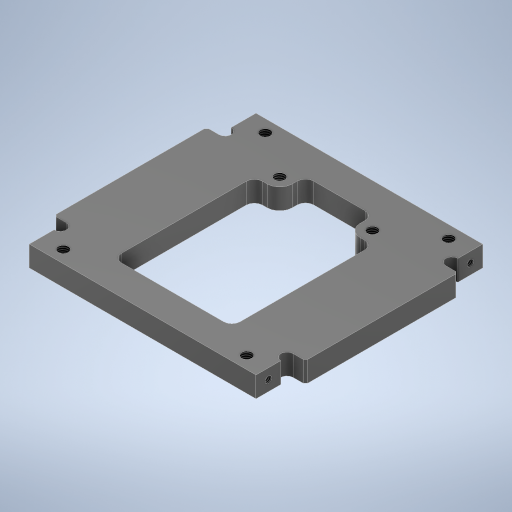
# Autodesk Inventor part: HeadUpperFrame
Saved by Autodesk Inventor 2024.2 (Build 282272000, 272)
## iProperties
Created: 2024-06-11
Part Number: HeadUpperFrame
Material: Acetal Resin, Black
Document SubType Name: Modeling
Designer: Masato Kubotera
Density: 1.425 g/cm^3
Appearance: Smooth - Black
Author: Masato Kubotera
Autodesk Inventor part; units mm, degrees
ref_plane "YZ Plane" through (0, 0, 0) normal (1, 0, 0) x (0, 1, 0)
ref_plane "XZ Plane" through (0, 0, 0) normal (0, 1, 0) x (-1, 0, 0)
ref_plane "XY Plane" through (0, 0, 0) normal (0, 0, 1) x (1, 0, 0)
sketch "Sketch1" plane through (0, 0, 0) normal (0, 0, 1) x (1, 0, 0)
  line L0 (-27.5, -27.5) -> (27.5, -27.5)
  line L1 (27.5, -27.5) -> (27.5, 27.5)
  line L2 (27.5, 27.5) -> (-27.5, 27.5)
  line L3 (-27.5, 27.5) -> (-27.5, -27.5)
  line L4 (-27.5, -27.5) -> (27.5, 27.5) construction
  line L5 (27.5, -27.5) -> (-27.5, 27.5) construction
  line L6 (-20, 14.15) -> (20, 14.15) construction
  line L7 (20, 14.15) -> (20, -14.15) construction
  line L8 (20, -14.15) -> (-20, -14.15) construction
  line L9 (-20, -14.15) -> (-20, 14.15) construction
  line L10 (-20, 14.15) -> (20, -14.15) construction
  line L11 (20, 14.15) -> (-20, -14.15) construction
  line L12 (0, -27.5) -> (0, 27.5) construction
  line L13 (-27.5, 0) -> (27.5, 0)
  line L14 (17, 11.25) -> (-17, 11.25) construction
  line L15 (-17, 11.25) -> (-17, -11.25) construction
  line L16 (-17, -11.25) -> (17, -11.25) construction
  line L17 (17, -11.25) -> (17, 11.25) construction
  line L18 (17, 11.25) -> (-17, -11.25) construction
  line L19 (-17, 11.25) -> (17, -11.25) construction
  line L20 (20.25, -12.4) -> (20.25, 12.4)
  line L21 (-18.5, -27.5) -> (-18.5, -30.5)
  line L22 (-18.5, -30.5) -> (18.5, -30.5)
  line L23 (18.5, -30.5) -> (18.5, -27.5)
  arc A0 (-18.5, -27.5) -> (-21.5, -27.5) centre (-20, -27.5) ccw
  line L24 (-24.5, -27.5) -> (-24.5, -21.5) construction
  arc A1 (21.5, -27.5) -> (18.5, -27.5) centre (20, -27.5) ccw
  line L25 (24.5, -27.5) -> (24.5, -21.5) construction
  line L26 (-18.5, 27.5) -> (-18.5, 30.5)
  line L27 (-18.5, 30.5) -> (18.5, 30.5)
  line L28 (18.5, 30.5) -> (18.5, 27.5)
  arc A2 (-21.5, 27.5) -> (-18.5, 27.5) centre (-20, 27.5) ccw
  line L29 (-24.5, 27.5) -> (-24.5, 21.5) construction
  arc A3 (18.5, 27.5) -> (21.5, 27.5) centre (20, 27.5) ccw
  line L30 (24.5, 27.5) -> (24.5, 21.5) construction
  line L31 (-12, -14.4) -> (18.25, -14.4)
  line L32 (-14, -12.4) -> (-14, -11.25)
  line L33 (-18.25, -8.25) -> (-17, -8.25)
  line L34 (-20.25, -6.25) -> (-20.25, 6.25)
  arc A4 (-14, -11.25) -> (-17, -8.25) centre (-17, -11.25) ccw
  line L35 (-12, 14.4) -> (18.25, 14.4)
  line L36 (-14, 12.4) -> (-14, 11.25)
  line L37 (-18.25, 8.25) -> (-17, 8.25)
  arc A5 (-17, 8.25) -> (-14, 11.25) centre (-17, 11.25) ccw
  arc A6 (-20.25, -6.25) -> (-18.25, -8.25) centre (-18.25, -6.25) ccw
  arc A7 (-14, -12.4) -> (-12, -14.4) centre (-12, -12.4) ccw
  arc A8 (18.25, -14.4) -> (20.25, -12.4) centre (18.25, -12.4) ccw
  arc A9 (20.25, 12.4) -> (18.25, 14.4) centre (18.25, 12.4) ccw
  arc A10 (-12, 14.4) -> (-14, 12.4) centre (-12, 12.4) ccw
  arc A11 (-18.25, 8.25) -> (-20.25, 6.25) centre (-18.25, 6.25) ccw
  line L38 (24.5, 22.25) -> (-24.5, 22.25) construction
  line L39 (-24.5, 22.25) -> (-24.5, -22.25) construction
  line L40 (-24.5, -22.25) -> (24.5, -22.25) construction
  line L41 (24.5, -22.25) -> (24.5, 22.25) construction
  line L42 (24.5, 22.25) -> (-24.5, -22.25) construction
  line L43 (-24.5, 22.25) -> (24.5, -22.25) construction
  line L44 (32.5, 26.5) -> (-32.5, 26.5) construction
  line L45 (-32.5, 26.5) -> (-32.5, -26.5) construction
  line L46 (-32.5, -26.5) -> (32.5, -26.5) construction
  line L47 (32.5, -26.5) -> (32.5, 26.5) construction
  line L48 (32.5, 26.5) -> (-32.5, -26.5) construction
  line L49 (-32.5, 26.5) -> (32.5, -26.5) construction
  circle A12 centre (-24.5, -22.25) radius 1.5 construction
  point P0 (0, 0)
  point P1 (21.5, 27.5)
  point P2 (-21.5, 27.5)
  point P3 (21.5, -27.5)
  point P4 (20.25, 0)
  point P5 (-14, -14.4)
  point P6 (20.25, -14.4)
  point P7 (-20.25, -8.25)
  point P8 (-14, 14.4)
  point P9 (20.25, 14.4)
  point P10 (-20.25, 8.25)
  point P11 (-20.25, 0)
  dimension "d0" = 55
  dimension "d1" = 55
  dimension "d2" = 40
  dimension "d3" = 28.3
  dimension "d4" = 34
  dimension "d5" = 22.5
  dimension "d8" = 1.5
  dimension "d9" = 6
  dimension "d10" = 6
  dimension "d11" = 3
  dimension "d35" = 6
  dimension "d36" = 0.25
  dimension "d37" = 0.25
  dimension "d38" = 2
  dimension "d39" = 6
  dimension "d40" = 8.5
  dimension "d41" = 16
  dimension "d42" = 1
  dimension "d43" = 3
  dimension "d44" = 3.75
  dimension "d45" = 49
  constraints: 100 end point, 24 point on circle, 23 symmetric about line, 17 point on line, 14 midpoint, 14 tangent, 13 centre point, 10 parallel, 8 coincident, 8 horizontal, 5 equal radius, 5 perpendicular, 5 vertical, 6 other
  measures "d0" distance of L2.end L1.end
  measures "d1" distance of L1.end L0.end
  measures "d2" distance of L7.end L8.end
  measures "d3" distance of L6.end L7.end
  measures "d4" distance of L16.end L15.end
  measures "d5" distance of L15.end L14.end
  measures "d8" radius of A0
  measures "d9" distance of L24.start L24.end
  measures "d10" distance of A0.end L0.start
  measures "d11" distance of L21.start L21.end
  measures "d35" diameter of A4
  measures "d36" distance between parallel lines of L31 L8
  measures "d37" distance between parallel lines of L9 L34
  measures "d38" radius of A6
  measures "d39" diameter of L3 L39
  measures "d40" diameter of L46 L40
  measures "d41" diameter of L45 L39
  measures "d42" distance between parallel lines of L0 L46
  measures "d43" diameter of A12
  measures "d44" distance edge to line of A12 L0
  measures "d45" distance of L38.start L38.end
extrude "Extrusion1" add sketch "Sketch1" along normal blind 5 contours L3 L13 L34 A6 L33 A4 L32 A7 L31 A8 L20 L1 L0 A1 A0 | L0 L23 L22 L21
hole "M3" at (-17, -11.25, 0) at (-24.5, -22.25, 0) at (24.5, -22.25, 0) direction (0, 0, 1) diameter 2.459 end through all thread size "M3x0.5" class "6H" standard "ANSI Metric M Profile"
sketch "Sketch2" plane through (21.5, -27.5, 0) normal (0, -1, 0) x (1, 0, 0)
  line L0 (3, 0) -> (3, 5)
  line L1 (-49, 5) -> (6, 5) projected
  line L2 (-46, 0) -> (-46, 5)
  line L3 (-49, 5) -> (6, 5) projected
  line L4 (0, 0) -> (6, 0) projected
  line L5 (-49, 0) -> (-43, 0) projected
  point P0 (0, 5)
  point P1 (-43, 5)
  point P2 (-46, 2.5)
  point P3 (3, 2.5)
  point P4 (3, 0)
  point P5 (3, 0)
  point P6 (3, 0)
  constraints: 4 end point, 4 midpoint, 2 point on line, 2 vertical
hole "Side-M2-6" at (24.5, -27.5, 2.5) at (-24.5, -27.5, 2.5) direction (0, 1, 0) diameter 1.567 depth 6 thread size "M2x0.4" class "6H" standard "ANSI Metric M Profile"
chamfer "C0.5" distance 0.5 angle 45 2 edges at (-18.5, -30.5, 2.5) (18.5, -30.5, 2.5)
mirror "Mirror1" about plane through (0, 0, 0) normal (0, 1, 0)
equation "\"d37\" = d36"
equation "\"d26\" = d9"
body "Solid1"
